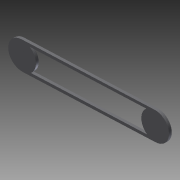
# Autodesk Inventor part: shooter elevation change proxy chain
Saved by Autodesk Inventor 2011 SP1 (Build 150282100, 282)
## iProperties
Created: 2012-01-20
Part Number: shooter elevation change proxy chain
Document SubType Name: Modeling
Designer: Christopher
Density: 1 g/cm^3
Author: Christopher
Autodesk Inventor part; units mm, degrees
ref_plane "YZ Plane" through (0, 0, 0) normal (1, 0, 0) x (0, 1, 0)
ref_plane "XZ Plane" through (0, 0, 0) normal (0, 1, 0) x (-1, 0, 0)
ref_plane "XY Plane" through (0, 0, 0) normal (0, 0, 1) x (1, 0, 0)
sketch "Sketch1" plane through (0, 0, 0) normal (0, 0, 1) x (1, 0, 0)
  circle A0 centre (-36.9883, -1.3696) radius 31.75
  circle A1 centre (267.8117, 11.3304) radius 31.75
  line L0 (-36.9883, 30.3804) -> (269.9527, 43.0081)
  line L1 (267.8117, -20.4196) -> (-35.6637, -33.0919)
  line L2 (-16.7002, -25.792) -> (249.593, -14.6723)
  line L3 (-18.9617, 24.7667) -> (247.4947, 35.7288)
  line L4 (-16.7002, -25.792) -> (-35.6637, -33.0919)
  line L5 (-18.9617, 24.7667) -> (-36.9883, 30.3804)
  line L6 (247.4947, 35.7288) -> (263.0758, 42.7252)
  line L7 (249.593, -14.6723) -> (267.8117, -20.4196)
  point P0 (0, 0)
  dimension "d0" = 12.7
  dimension "d1" = 304.8
  dimension "d2" = 63.5
  dimension "d3" = 63.5
  dimension "d4" = 6.35
  dimension "d5" = 6.5024
  constraints: 16 end point, 9 point on circle, 2 centre point, 2 parallel, 1 point on line, 1 tangent
  measures "d0" vertical distance of A0.centre A1.centre
  measures "d1" horizontal distance of A0.centre A1.centre
  measures "d2" diameter of A0
  measures "d3" diameter of A1
  measures "d4" distance between parallel lines of L0 L3
  measures "d5" distance between parallel lines of L1 L2
extrude "Extrusion1" add sketch "Sketch1" against normal blind 6.35 contours A0 L4 L5 | L5 A0 | A0 L0 A1 L3 | L2 A1 L1 A0 | A0 L4 | L6 L0 A1 L7 | A1 L6 | L7 A1
body "Solid1"
